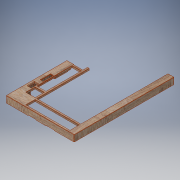
# Autodesk Inventor part: TopCase
Saved by Autodesk Inventor 2018 (Build 220112000, 112)
## iProperties
Created: 2024-10-01
Part Number: TopCase
Material: Wood (Maple)
Document SubType Name: Modeling
Designer: yuchi
Density: 0.67 g/cm^3
Appearance: Oak - Herringbone
Author: yuchi
Autodesk Inventor part; units mm, degrees
ref_plane "YZ Plane" through (0, 0, 0) normal (1, 0, 0) x (0, 1, 0)
sketch "Sketch2" plane through (0, 0, 0) normal (0, 1, 0) x (-1, 0, 0)
  line L0 (12.7, -3.9682) -> (152.454, -3.9682)
  line L1 (119.6499, -137.3179) -> (119.6499, -146.8429)
  line L2 (119.6499, -146.8429) -> (95.8374, -146.8429)
  line L3 (95.8374, -146.8429) -> (95.8374, -156.3679)
  line L4 (95.8374, -156.3679) -> (76.7874, -156.3679)
  line L5 (76.7874, -156.3679) -> (76.7874, -161.1304)
  line L6 (76.7874, -161.1304) -> (57.7374, -161.1304)
  line L7 (57.7374, -161.1304) -> (57.7374, -170.6554)
  line L8 (57.7374, -170.6554) -> (38.6874, -170.6554)
  line L9 (38.6874, -170.6554) -> (38.6874, -223.0434)
  line L10 (12.7, -223.0434) -> (38.6874, -223.0434)
  line L11 (149.794, -46.2682) -> (142.144, -46.2682)
  line L12 (142.144, -46.2682) -> (142.144, -61.4382)
  line L13 (142.144, -61.4382) -> (149.794, -61.4382)
  line L14 (149.794, -61.4382) -> (149.794, -46.2682)
  line L15 (138.7, -32.5419) -> (119.65, -32.5419)
  line L16 (119.65, -32.5419) -> (119.65, -51.5919)
  line L17 (119.65, -51.5919) -> (138.7, -51.5919)
  line L18 (138.7, -51.5919) -> (138.7, -32.5419)
  line L19 (138.7, -56.3549) -> (119.65, -56.3549)
  line L20 (119.65, -56.3549) -> (119.65, -132.5549)
  line L21 (119.65, -132.5549) -> (138.7, -132.5549)
  line L22 (138.7, -132.5549) -> (138.7, -56.3549)
  line L23 (114.887, -32.5434) -> (114.887, -73.9353)
  line L24 (114.887, -73.9353) -> (114.887, -146.8429)
  line L25 (114.887, -32.5434) -> (19.637, -32.5434)
  line L26 (19.637, -32.5434) -> (19.637, -223.0434)
  line L27 (114.887, -27.7804) -> (19.637, -27.7804)
  line L28 (114.887, -27.7804) -> (114.887, -8.7304)
  line L29 (114.887, -8.7304) -> (19.637, -8.7304)
  line L30 (19.637, -8.7304) -> (19.637, -27.7804)
  line L31 (12.7, -3.9682) -> (7.183, -3.9682)
  line L32 (7.183, -223.0434) -> (12.7, -223.0434)
  line L33 (152.454, -3.9682) -> (152.7, -3.9682)
  line L34 (149.195, -71.4432) -> (143.445, -71.4432)
  line L35 (143.445, -71.4432) -> (143.445, -93.9432)
  line L36 (143.445, -93.9432) -> (149.195, -93.9432)
  line L37 (149.195, -93.9432) -> (149.195, -71.4432)
  line L38 (6.2, -3.9682) -> (7.183, -3.9682)
  line L39 (6.2, -3.9682) -> (6.2, -223.0434)
  line L40 (6.2, -223.0434) -> (7.183, -223.0434)
  line L41 (138.932, -51.9234) -> (119.4185, -51.9234)
  line L42 (138.932, -56.0234) -> (119.4185, -56.0234)
  line L43 (119.4185, -56.0234) -> (119.4185, -132.8864)
  line L44 (119.4185, -136.9864) -> (119.65, -136.9864)
  line L45 (119.4185, -136.9864) -> (119.4185, -146.8429)
  line L46 (138.932, -51.9234) -> (138.932, -32.2099)
  line L47 (138.932, -32.2099) -> (130.4516, -32.2099)
  line L48 (130.4516, -32.2099) -> (119.4185, -32.2099)
  line L49 (119.4185, -32.2099) -> (119.4185, -51.9234)
  line L50 (138.932, -56.0234) -> (138.932, -132.8864)
  line L51 (138.932, -132.8864) -> (119.4185, -132.8864)
  line L52 (115.119, -28.1119) -> (19.405, -28.1119)
  line L53 (115.1185, -32.2119) -> (19.405, -32.2119)
  line L54 (19.405, -28.1119) -> (19.405, -8.3984)
  line L55 (115.119, -28.1119) -> (115.119, -8.3984)
  line L56 (115.119, -8.3984) -> (19.405, -8.3984)
  line L57 (115.1185, -32.2119) -> (115.1185, -146.8429)
  line L58 (19.405, -32.2119) -> (19.405, -223.0434)
  line L59 (152.7, -3.9682) -> (154.2, -3.9682)
  line L60 (154.2, -3.9682) -> (154.2, -137.3179)
  line L61 (142.144, -46.2682) -> (142.144, -6.3492)
  line L62 (142.144, -6.3492) -> (12.7, -6.3492)
  line L63 (12.7, -6.3492) -> (12.7, -223.0434)
  line L64 (149.794, -61.4382) -> (152.7, -61.4382)
  line L65 (138.932, -136.9864) -> (138.932, -137.3179)
  line L66 (138.932, -136.9864) -> (119.65, -136.9864)
  line L67 (154.2, -137.3179) -> (119.6499, -137.3179)
  line L68 (138.932, -137.3179) -> (119.4185, -137.3179)
  line L69 (119.4185, -137.3179) -> (119.4185, -136.9864)
  line L70 (119.4185, -136.9864) -> (138.932, -136.9864)
  line L71 (138.932, -136.9864) -> (138.932, -137.3179)
  line L72 (119.4185, -146.8429) -> (119.6499, -146.8429)
  line L73 (119.6499, -146.8429) -> (119.6499, -137.3179)
  line L74 (119.6499, -137.3179) -> (119.4185, -137.3179)
  line L75 (119.4185, -137.3179) -> (119.4185, -146.8429)
  line L76 (119.6499, -146.8429) -> (119.4185, -146.8429)
  line L77 (119.4185, -146.8429) -> (119.4185, -137.3179)
  line L78 (119.4185, -137.3179) -> (119.6499, -137.3179)
  line L79 (119.6499, -137.3179) -> (119.6499, -146.8429)
  line L80 (152.7, -61.4382) -> (152.7, -137.3179)
  line L81 (152.7, -137.3179) -> (138.932, -137.3179)
  line L82 (138.932, -136.9864) -> (138.932, -137.3179)
  line L83 (138.932, -136.9864) -> (119.4185, -136.9864)
  line L84 (119.4185, -136.9864) -> (119.4185, -146.8429)
  line L85 (119.4185, -146.8429) -> (115.1185, -146.8429)
  line L86 (115.1185, -146.8429) -> (115.1185, -32.2119)
  line L87 (115.1185, -32.2119) -> (19.405, -32.2119)
  line L88 (19.405, -32.2119) -> (19.405, -223.0434)
  line L89 (19.405, -223.0434) -> (12.7, -223.0434)
  line L90 (12.7, -223.0434) -> (12.7, -6.3492)
  line L91 (12.548, -6.3492) -> (142.144, -6.3492)
  line L92 (142.144, -6.3492) -> (142.144, -46.2682)
  line L93 (142.144, -46.2682) -> (142.144, -61.4382)
  line L94 (142.144, -61.4382) -> (152.7, -61.4382)
  line L95 (147.054, -137.3179) -> (147.054, -101.4889)
  line L96 (147.054, -101.4889) -> (152.7, -101.4889)
  point P0 (0, 0)
  point P1 (152.454, -6.3489)
  point P2 (127.8231, -53.9734)
  point P3 (117.2685, -47.3899)
  point P4 (128.6114, -134.9364)
  point P5 (108.1778, -30.1619)
  point P6 (150.627, -127.3179)
  point P7 (9.45, -127.3179)
  point P8 (9.45, -212.9184)
  point P9 (9.45, -13.9682)
  point P10 (150.627, -13.9682)
  dimension "d32" = 9.525
  dimension "d33" = 23.8125
  dimension "d34" = 9.525
  dimension "d35" = 19.05
  dimension "d36" = 4.7625
  dimension "d37" = 19.05
  dimension "d38" = 9.525
  dimension "d39" = 19.05
  dimension "d40" = 52.388
  dimension "d45" = 15.17
  dimension "d51" = 19.05
  dimension "d52" = 76.2
  dimension "d53" = 4.763
  dimension "d55" = 4.763
  dimension "d56" = 19.05
  dimension "d60" = 0.246
  dimension "d65" = 10.005
  dimension "d66" = 22.5
  dimension "d68" = 13.754
  dimension "d75" = 5.75
  dimension "d80" = 2.66
  dimension "d82" = 2.3815
  dimension "d83" = 2.3815
  dimension "d84" = 2.05
  dimension "d85" = 2.05
  dimension "d86" = 2.3815
  dimension "d88" = 4.763
  dimension "d89" = 2.15
  dimension "d97" = 0.232
  dimension "d98" = 19.05
  dimension "d99" = 19.05
  dimension "d100" = 0.332
  dimension "d101" = 0.232
  dimension "d102" = 2.3815
  dimension "d103" = 2.05
  dimension "d104" = 2.05
  dimension "d105" = 0.232
  dimension "d106" = 0.232
  dimension "d107" = 0.332
  dimension "d108" = 2.15
  dimension "d109" = 0.232
  dimension "d113" = 1.5
  dimension "d132" = 35.829
  dimension "d144" = 7.146
  dimension "d145" = 3.573
  dimension "d146" = 10
  dimension "d147" = 3.25
  dimension "d149" = 3.25
  dimension "d150" = 3.573
  dimension "d151" = 10
  dimension "d153" = 10.125
  dimension "d157" = 10
  dimension "d158" = 10
  dimension "d180" = 3.25
  dimension "d221" = 130.9681
  dimension "d224" = 43.4216
  dimension "d275" = 4.763
  dimension "d276" = 148
  dimension "d277" = 95.25
  dimension "d278" = 95.25
  dimension "d279" = 190.5
  constraints: 194 end point, 27 perpendicular, 26 horizontal, 22 parallel, 12 vertical, 11 point on line, 6 collinear
  measures "d32" distance of L1.start L1.end
  measures "d33" distance of L1.end L2.end
  measures "d34" distance of L2.end L3.end
  measures "d35" distance of L3.end L4.end
  measures "d36" distance of L4.end L5.end
  measures "d37" distance of L5.end L6.end
  measures "d38" distance of L6.end L7.end
  measures "d39" distance of L7.end L8.end
  measures "d40" distance of L8.end L9.end
  measures "d45" distance between parallel lines of L13 L11
  measures "d51" distance of L20.end L21.end
  measures "d52" distance of L19.end L20.end
  measures "d53" distance between parallel lines of L16 L23
  measures "d55" distance between parallel lines of L27 L25
  measures "d56" distance of L27.start L28.end
  measures "d60" distance of L0.end L33.end
  measures "d65" distance between parallel lines of L13 L34
  measures "d66" distance between parallel lines of L36 L34
  measures "d68" distance from line of point (152.454, -6.349) L18
  measures "d75" distance between parallel lines of L35 L37
  measures "d80" distance from line of point (152.454, -6.349) L14
  measures "d82" distance from line of L17 point (127.823, -53.973)
  measures "d83" distance from line of L19 point (127.823, -53.973)
  measures "d84" distance from line of L41 point (127.823, -53.973)
  measures "d85" distance from line of point (127.823, -53.973) L42
  measures "d86" distance from line of L23 point (117.269, -47.39)
  measures "d88" distance between parallel lines of L20 L23
  measures "d89" distance from line of L43 point (117.269, -47.39)
  measures "d97" distance from line of L41.start L18
  measures "d98" distance between parallel lines of L16 L18
  measures "d99" distance between parallel lines of L17 L15
  measures "d100" distance from line of L15 L46.end
  measures "d101" distance from line of L42.start L22
  measures "d102" distance from line of L25 point (108.178, -30.162)
  measures "d103" distance from line of L52 point (108.178, -30.162)
  measures "d104" distance from line of L53 point (108.178, -30.162)
  measures "d105" distance from line of L30 L52.end
  measures "d106" distance between parallel lines of L55 L28
  measures "d107" distance between parallel lines of L56 L29
  measures "d108" horizontal distance of L53.start point (117.269, -47.39)
  measures "d109" distance between parallel lines of L26 L58
  measures "d113" distance of L33.end L59.end
  measures "d132" distance of L95.start L95.end
  measures "d144" distance between parallel lines of L60 L95
  measures "d145" distance from line of L95 point (150.627, -127.318)
  measures "d146" distance from line of L31 point (9.45, -13.968)
  measures "d147" distance from line of L39 point (9.45, -13.968)
  measures "d149" distance from line of L39 point (9.45, -212.918)
  measures "d150" distance from line of L60 point (150.627, -13.968)
  measures "d151" distance from line of L0 point (150.627, -13.968)
  measures "d153" distance from line of L32 point (9.45, -212.918)
  measures "d157" distance from line of L67 point (150.627, -127.318)
  measures "d158" distance from line of point (9.45, -127.318) L81
  measures "d180" distance from line of L39 point (9.45, -127.318)
  measures "d221" distance from line of point (128.611, -134.936) L33
  measures "d224" distance from line of point (117.269, -47.39) L33
  measures "d275" distance between parallel lines of L16 L28
  measures "d276" distance between parallel lines of L39 L60
  measures "d277" distance between parallel lines of L23 L26
  measures "d278" distance between parallel lines of L30 L28
  measures "d279" distance between parallel lines of L25 L10
extrude "Extrusion5" add sketch "Sketch2" along normal blind 14 contours L0 L33 L59 L60 L67 L80 L64 L14 L11 L61 L62 L63 L32 L40 L39 L38 L31 | L67 L95 L96 L80 | L63 L62 L61 L12 L13 L64 L80 L96 L95 L67 L65 L66 L44 L45 L2 L57 L53 L58 L10 | L67 L68 L45 L44 L66 L65 | L1 L2 L45 L68
extrude "Extrusion6" cut sketch "Sketch2" along normal blind 14 contours L67 L68 L45 L44 L66 L65
extrude "Extrusion7" cut sketch "Sketch2" along normal blind 14 contours L1 L2 L45 L68
extrude "Extrusion8" cut sketch "Sketch2" along normal blind 10.3 contours L67 L95 L96 L80 | L63 L62 L61 L12 L13 L64 L80 L96 L95 L67 L65 L66 L44 L45 L2 L57 L53 L58 L10 | L13 L12 L11 L14 | L18 L17 L16 L15 | L22 L21 L20 L19 | L27 L30 L29 L28 | L37 L36 L35 L34 | L41 L49 L48 L47 L46 | L50 L51 L43 L42 | L52 L54 L56 L55
extrude "Extrusion9" add sketch "Sketch2" along normal blind 10.3 contours L67 L95 L96 L80
sketch "Sketch8" plane through (-154.2, 0, -137.3179) normal (-1, 0, 0) x (0, 0, 1)
  line L0 (0, 0) -> (0, 14) projected
  line L1 (133.3496, 0) -> (0, 0)
  line L2 (0, 0) -> (0, 14)
  line L3 (0, 14) -> (133.3496, 14)
  line L4 (133.3496, 14) -> (133.3496, 0)
  point P0 (137.3179, 0)
  constraints: 8 end point, 2 parallel, 1 horizontal, 1 perpendicular
extrude "Extrusion10" cut sketch "Sketch8" against normal blind 0.268
sketch "Sketch9" plane through (-6.2, 0, -3.9682) normal (1, 0, 0) x (0, 0, -1)
  line L0 (133.3496, 14) -> (0, 14) projected
  line L1 (2.381, 0) -> (219.0751, 0) projected
  line L2 (0, 14) -> (219.0751, 14)
  line L3 (219.0751, 14) -> (219.0751, 0)
  line L4 (219.0751, 0) -> (0, 0)
  line L5 (0, 0) -> (0, 14)
  point P0 (-3.9682, 0)
  constraints: 8 end point, 2 parallel, 1 horizontal, 1 perpendicular
extrude "Extrusion11" cut sketch "Sketch9" against normal blind 0.049
sketch "Sketch10" plane through (-19.405, 14, -223.0434) normal (-1, 0, 0) x (0, 0, 1)
  line L0 (0, 0) -> (190.8315, 0) projected
  line L1 (216.6941, -3.7) -> (0, -3.7) projected
  line L2 (190.8315, 0) -> (0, 0)
  line L3 (0, 0) -> (0, -3.7)
  line L4 (0, -3.7) -> (190.8315, -3.7)
  line L5 (190.8315, -3.7) -> (190.8315, 0)
  point P0 (223.0434, -14)
  constraints: 8 end point, 2 parallel, 1 horizontal, 1 perpendicular
extrude "Extrusion12" cut sketch "Sketch10" against normal blind 0.473
sketch "Sketch11" plane through (-19.405, 14, -28.1119) normal (-1, 0, 0) x (0, 0, 1)
  line L0 (0, -3.7) -> (19.7135, -3.7) projected
  line L1 (19.7135, 0) -> (0, 0)
  line L2 (0, 0) -> (0, -3.7)
  line L3 (0, -3.7) -> (19.7135, -3.7)
  line L4 (19.7135, -3.7) -> (19.7135, 0)
  point P0 (28.1119, -14)
  constraints: 8 end point, 2 parallel, 1 horizontal, 1 perpendicular
extrude "Extrusion13" cut sketch "Sketch11" against normal blind 0.473
hole "Hole1" at (-9.45, 0, -127.3179) at (-9.45, 0, -212.9184) at (-9.45, 0, -13.9682) direction (0, 1, 0) diameter 2 depth 10 tip angle 118
chamfer "Chamfer2" distance 0.5 angle 45 22 edges at (-18.932, 14, -127.6276) (-67.0255, 14, -28.1119) (-67.0253, 14, -32.2119) (-18.932, 14, -18.2551) (-67.0255, 14, -8.3984) (-115.119, 14, -18.2551) (-129.1753, 14, -32.2099) (-138.932, 14, -42.0666) (-119.4185, 14, -42.0666) (-129.1753, 14, -51.9234) (-142.144, 14, -53.8532) (-145.969, 14, -46.2682) (-149.794, 14, -53.8532) (-145.969, 14, -61.4382) (-129.1753, 14, -56.0234) (-138.932, 14, -94.4549) (-119.4185, 14, -94.4549) (-129.1753, 14, -132.8864) (-115.1185, 14, -89.5274) (-129.1753, 14, -136.9864) (-119.4185, 14, -141.9146) (-138.932, 14, -137.1521)
sketch "Sketch13" plane through (-12.7, 0, -6.3492) normal (-1, 0, 0) x (0, 0, 1)
  line L0 (0, 0) -> (0, 10.3) projected
  line L1 (-216.6941, 0) -> (-216.6941, 10.3) projected
  line L2 (0, 10.3) -> (-216.6941, 10.3)
  line L3 (-216.6941, 10.3) -> (-216.6941, 0)
  line L4 (-216.6941, 0) -> (0, 0)
  line L5 (0, 0) -> (0, 10.3)
  point P0 (6.3492, 0)
  constraints: 8 end point, 2 parallel, 1 horizontal, 1 perpendicular
extrude "Extrusion14" cut sketch "Sketch13" against normal blind 0.268
sketch "Sketch14" plane through (-12.432, 0, -6.3492) normal (-1, 0, 0) x (0, 0, 1)
  line L0 (0, 0) -> (-216.6941, 0) projected
  line L1 (0, 10.3) -> (-20, 10.3)
  line L2 (-20, 10.3) -> (-20, 0)
  line L3 (-20, 0) -> (0, 0)
  line L4 (0, 0) -> (0, 10.3)
  line L5 (-216.6941, 10.3) -> (-196.6941, 10.3)
  line L6 (-196.6941, 10.3) -> (-196.6941, 0)
  line L7 (-196.6941, 0) -> (-216.6941, 0)
  line L8 (-216.6941, 0) -> (-216.6941, 10.3)
  line L9 (-216.6941, 10.3) -> (0, 10.3) projected
  line L10 (-100.9681, 10.3) -> (-140.9681, 10.3)
  line L11 (-140.9681, 10.3) -> (-140.9681, 0)
  line L12 (-140.9681, 0) -> (-100.9681, 0)
  line L13 (-100.9681, 0) -> (-100.9681, 10.3)
  line L14 (-20, 10.3) -> (-100.9681, 10.3)
  line L15 (-100.9681, 10.3) -> (-100.9681, 0)
  line L16 (-100.9681, 0) -> (-20, 0)
  line L17 (-20, 0) -> (-20, 10.3)
  line L18 (-140.9681, 10.3) -> (-196.6941, 10.3)
  line L19 (-196.6941, 10.3) -> (-196.6941, 0)
  line L20 (-196.6941, 0) -> (-140.9681, 0)
  line L21 (-140.9681, 0) -> (-140.9681, 10.3)
  point P0 (6.3492, 0)
  dimension "d183" = 20
  dimension "d184" = 20
  dimension "d185" = 75.726
  dimension "d186" = 115.726
  constraints: 40 end point, 10 parallel, 5 horizontal, 5 perpendicular, 4 point on line
  measures "d183" distance of L3.end L2.end
  measures "d184" distance of L6.end L7.end
  measures "d185" distance between parallel lines of L11 L8
  measures "d186" distance between parallel lines of L13 L8
extrude "Extrusion16" cut sketch "Sketch14" against normal blind 3.25 contours L0 L13 L9 L2 | L0 L6 L9 L11
sketch "Sketch16" plane through (0, 0, 0) normal (0, -1, 0) x (1, 0, 0)
  line L0 (-142.144, -35.1182) -> (-146.144, -35.1182)
  line L1 (-146.144, -35.1182) -> (-146.144, -15.1182)
  line L2 (-146.144, -15.1182) -> (-142.144, -15.1182)
  line L3 (-142.144, -15.1182) -> (-142.144, -35.1182)
  line L4 (-153.932, -3.9682) -> (-6.249, -3.9682) projected
  point P0 (0, 0)
  point P1 (-142.144, -46.2682)
  point P2 (-152.932, -3.9682)
  point P3 (-7.249, -3.9683)
  dimension "d195" = 4
  dimension "d196" = 20
  dimension "d197" = 11.15
  constraints: 8 end point, 3 perpendicular, 1 horizontal
  measures "d195" distance of L0.start L0.end
  measures "d196" distance of L0.end L1.end
  measures "d197" distance between parallel lines of L4 L2
extrude "Extrusion17" cut sketch "Sketch16" against normal blind 10.3
fillet "Fillet6" radius 1 1 edges at (-12.432, 5.15, -6.3492)
sketch "Sketch18" plane through (-152.7, 0, -101.4889) normal (0, 0, 1) x (1, 0, 0)
  line L0 (0, 10.3) -> (5.646, 10.3) projected
  line L1 (5.646, 10.3) -> (0, 10.3)
  line L2 (0, 10.3) -> (0, 0)
  line L3 (0, 0) -> (5.646, 0)
  line L4 (5.646, 0) -> (5.646, 10.3)
  point P0 (152.7, 0)
  constraints: 8 end point, 2 parallel, 1 horizontal, 1 perpendicular
extrude "Extrusion18" cut sketch "Sketch18" against normal blind 1
sketch "Sketch19" plane through (-147.054, 0, -137.3179) normal (1, 0, 0) x (0, 0, -1)
  line L0 (0, 10.3) -> (-34.829, 10.3)
  line L1 (-34.829, 10.3) -> (-34.829, 0)
  line L2 (-34.829, 0) -> (0, 0)
  line L3 (0, 0) -> (0, 10.3)
  point P0 (-137.3179, 0)
  constraints: 8 end point, 2 parallel, 1 horizontal, 1 perpendicular
extrude "Extrusion19" add sketch "Sketch19" against normal blind 4
sketch "Sketch20" plane through (0, 0, 0) normal (0, -1, 0) x (1, 0, 0)
  line L0 (-147.054, -137.3179) -> (-153.932, -137.3179) projected
  line L1 (-153.932, -3.9682) -> (-153.932, -137.3179) projected
  line L2 (-153.932, -3.9682) -> (-6.249, -3.9682) projected
  point P0 (0, 0)
  point P1 (-150.432, -127.3179)
  point P2 (-150.432, -13.9682)
  point P3 (-142.932, -137.3179)
  point P4 (-153.932, -4.9682)
  point P5 (-152.932, -3.9682)
  point P6 (-7.249, -3.9683)
  dimension "d236" = 10
  dimension "d237" = 3.5
  dimension "d238" = 3.5
  dimension "d239" = 10
  measures "d236" distance from line of point (-150.432, -127.318) L0
  measures "d237" distance from line of L1 point (-150.432, -127.318)
  measures "d238" distance from line of L1 point (-150.432, -13.968)
  measures "d239" distance from line of L2 point (-150.432, -13.968)
hole "Hole3" at (-150.432, 0, -127.3179) at (-150.432, 0, -13.9682) direction (0, 1, 0) diameter 2 depth 10 tip angle 118
sketch "Sketch21" plane through (0, 0, 0) normal (0, -1, 0) x (1, 0, 0)
  line L0 (-153.932, -3.9682) -> (-153.932, -137.3179) projected
  line L1 (-147.054, -102.4889) -> (-152.7, -102.4889) projected
  line L2 (-6.249, -223.0434) -> (-6.249, -3.9682) projected
  circle A0 centre (-149.932, -122.3179) radius 0.75
  circle A1 centre (-9.95, -122.3179) radius 0.75
  line L3 (-153.932, -3.9682) -> (-6.249, -3.9682) projected
  circle A2 centre (-149.932, -8.9682) radius 0.75
  line L4 (-9.182, -203.0434) -> (-12.432, -203.0434) projected
  circle A3 centre (-9.95, -207.9184) radius 0.75
  line L5 (-147.054, -137.3179) -> (-153.932, -137.3179) projected
  circle A4 centre (-150.432, -127.3179) radius 1 projected
  circle A5 centre (-150.432, -13.9682) radius 1 projected
  circle A6 centre (-9.45, -127.3179) radius 1 projected
  line L6 (-9.182, -107.3174) -> (-12.432, -107.3174) projected
  circle A7 centre (-9.45, -212.9184) radius 1 projected
  point P0 (0, 0)
  point P1 (-153.932, -4.9682)
  point P2 (-149.054, -102.4889)
  point P3 (-6.249, -4.9683)
  point P4 (-152.932, -3.9682)
  point P5 (-7.249, -3.9683)
  point P6 (-10.182, -203.0434)
  point P7 (-11.432, -203.0434)
  point P8 (-10.182, -107.3174)
  point P9 (-11.432, -107.3174)
  dimension "d252" = 1.5
  dimension "d253" = 1.5
  dimension "d255" = 1.5
  dimension "d259" = 1.5
  dimension "d270" = 0.5
  dimension "d273" = 5
  dimension "d274" = 0.5
  dimension "d291" = 0.5
  dimension "d333" = 5
  dimension "d335" = 5
  dimension "d347" = 5
  dimension "d348" = 0.5
  constraints: 8 coincident, 4 centre point
  measures "d252" diameter of A0
  measures "d253" diameter of A1
  measures "d255" diameter of A2
  measures "d259" diameter of A3
  measures "d270" horizontal distance of point (-150.432, -127.318) point (-149.932, -122.318)
  measures "d273" vertical distance of point (-149.932, -8.968) point (-150.432, -13.968)
  measures "d274" horizontal distance of A2.centre point (-150.432, -13.968)
  measures "d291" horizontal distance of point (-9.95, -122.318) point (-9.45, -127.318)
  measures "d333" vertical distance of point (-149.932, -122.318) point (-150.432, -127.318)
  measures "d335" vertical distance of point (-9.45, -127.318) point (-9.95, -122.318)
  measures "d347" vertical distance of point (-9.95, -207.918) point (-9.45, -212.918)
  measures "d348" horizontal distance of A3.centre point (-9.45, -212.918)
hole "Hole4" at (-149.932, 0, -122.3179) at (-9.95, 0, -122.3179) at (-149.932, 0, -8.9682) at (-9.95, 0, -207.9184) direction (0, 1, 0) diameter 2 depth 10 tip angle 118
sketch "Sketch25" plane through (-6.249, 0, -3.9682) normal (1, 0, 0) x (0, 0, -1)
  line L0 (3.381, 0) -> (219.0751, 0) projected
  line L1 (0, 14) -> (0, 0) projected
  line L2 (219.0751, 0) -> (0, 0)
  line L3 (0, 0) -> (0, 14)
  line L4 (0, 14) -> (219.0751, 14)
  line L5 (219.0751, 14) -> (219.0751, 0)
  point P0 (-3.9682, 0)
  point P1 (200.0751, 0)
  constraints: 8 end point, 2 parallel, 1 horizontal, 1 perpendicular
extrude "Extrusion20" add sketch "Sketch25" along normal blind 0.817
sketch "Sketch27" plane through (-147.054, 0, -137.3179) normal (1, 0, 0) x (0, 0, -1)
  line L0 (-34.829, 10.3) -> (0, 10.3) projected
  line L1 (-34.829, 10.3) -> (-34.829, 0) projected
  line L2 (0, 10.3) -> (-34.829, 10.3)
  line L3 (-34.829, 10.3) -> (-34.829, 0)
  line L4 (-34.829, 0) -> (0, 0)
  line L5 (0, 0) -> (0, 10.3)
  point P0 (-137.3179, 0)
  constraints: 8 end point, 2 parallel, 1 horizontal, 1 perpendicular
extrude "Extrusion21" cut sketch "Sketch27" against normal blind 1.378
sketch "Sketch33" plane through (-153.932, 0, -137.3179) normal (-1, 0, 0) x (0, 0, 1)
  line L0 (0, 14) -> (133.3496, 14) projected
  line L1 (0, 10.3) -> (0, 0) projected
  line L2 (133.3496, 14) -> (0, 14)
  line L3 (0, 14) -> (0, 0)
  line L4 (0, 0) -> (133.3496, 0)
  line L5 (133.3496, 0) -> (133.3496, 14)
  point P0 (137.3179, 0)
  constraints: 8 end point, 2 parallel, 1 horizontal, 1 perpendicular
extrude "Extrusion26" add sketch "Sketch33" along normal blind 1
ref_plane "Work Plane5" through (-153.932, 13.5, -3.9682) normal (0, 0, 1) x (1, 0, 0)
sketch "Sketch34" plane through (-153.932, 13.5, -3.9682) normal (0, 0, 1) x (1, 0, 0)
  line L0 (148.5, -13.5) -> (148.5, 0) projected
  line L1 (-1, -13.5) -> (148.5, -13.5) projected
  arc A0 (89.129, -12.466) -> (89.129, -19.566) centre (89.129, -16.016) ccw
  arc A1 (103.149, -19.566) -> (103.149, -12.466) centre (103.149, -16.016) ccw
  line L2 (89.129, -12.466) -> (103.149, -12.466)
  line L3 (103.149, -19.566) -> (89.129, -19.566)
  arc A2 (63.269, -19.566) -> (63.269, -12.466) centre (63.269, -16.016) ccw
  arc A3 (49.249, -12.466) -> (49.249, -19.566) centre (49.249, -16.016) ccw
  line L4 (49.249, -19.566) -> (63.269, -19.566)
  line L5 (63.269, -12.466) -> (49.249, -12.466)
  point P0 (153.932, -13.5)
  point P1 (96.139, -16.016)
  point P2 (0, -13.5)
  point P3 (147.5, -13.5)
  point P4 (56.259, -16.016)
  dimension "d315" = 2.516
  dimension "d316" = 52.361
  dimension "d317" = 39.88
  dimension "d318" = 2.516
  dimension "d319" = 7.01
  dimension "d320" = 7.01
  dimension "d321" = 7.01
  dimension "d322" = 7.01
  dimension "d323" = 3.55
  dimension "d324" = 3.55
  dimension "d325" = 3.55
  dimension "d326" = 3.55
  dimension "d327" = 7.1
  dimension "d328" = 7.1
  constraints: 8 end point, 8 point on circle, 4 centre point, 4 coincident, 4 horizontal alignment, 2 horizontal, 2 parallel, 1 tangent
  measures "d315" distance from line of L1 point (96.139, -16.016)
  measures "d316" distance from line of L0 point (96.139, -16.016)
  measures "d317" distance of point (96.139, -16.016) point (56.259, -16.016)
  measures "d318" distance from line of L1 point (56.259, -16.016)
  measures "d319" distance of point (63.269, -16.016) point (56.259, -16.016)
  measures "d320" distance of point (56.259, -16.016) point (49.249, -16.016)
  measures "d321" distance of point (96.139, -16.016) point (89.129, -16.016)
  measures "d322" distance of point (103.149, -16.016) point (96.139, -16.016)
  measures "d323" radius of A0
  measures "d324" radius of A1
  measures "d325" radius of A2
  measures "d326" radius of A3
  measures "d327" distance between parallel lines of L4 L5
  measures "d328" distance between parallel lines of L2 L3
extrude "Extrusion27" cut sketch "Sketch34" against normal blind 10
sketch "Sketch35" plane through (-138.932, 10.3, -137.3179) normal (0, 0, -1) x (-1, 0, 0)
  line L0 (9.5, -10.3) -> (16, -10.3) projected
  line L1 (16, 3.7) -> (16, -10.3) projected
  line L2 (10.862, -10.3) -> (3.212, -10.3) projected
  line L3 (3.212, -10.3) -> (-125.5, -10.3) projected
  arc A0 (11.6009, -10.3) -> (9.232, -9.394) centre (9.232, -12.944) ccw
  line L4 (2.212, -10.3) -> (3.212, -10.3) projected
  line L5 (11.6009, -10.3) -> (2.212, -10.3)
  line L6 (9.232, -9.394) -> (2.212, -9.394)
  line L7 (2.212, 0) -> (2.212, -10.3) projected
  line L8 (2.212, -10.3) -> (2.212, -9.394)
  point P0 (-138.932, -10.3)
  point P1 (2.222, -12.944)
  point P2 (16, 3.2)
  point P3 (4.212, -10.3)
  point P4 (-32.0237, -10.3)
  point P5 (-50.4943, -10.3)
  dimension "d336" = 2.644
  dimension "d337" = 13.778
  dimension "d338" = 7.01
  dimension "d342" = 3.55
  dimension "d343" = 3.55
  constraints: 6 end point, 2 collinear, 2 point on circle, 1 centre point, 1 coincident, 1 horizontal, 1 point on line
  measures "d336" distance from line of L0 point (2.222, -12.944)
  measures "d337" distance from line of L1 point (2.222, -12.944)
  measures "d338" distance of point (9.232, -12.944) point (2.222, -12.944)
  measures "d342" radius of A0
  measures "d343" distance from line of point (2.222, -12.944) L6
extrude "Extrusion28" cut sketch "Sketch35" against normal blind 6
sketch "Sketch37" plane through (0, 0, 0) normal (0, -1, 0) x (1, 0, 0)
  line L0 (-12.432, -7.3492) -> (-12.432, -5.9682)
  line L1 (-48.6007, -5.9682) -> (-13.432, -5.9682) projected
  line L2 (-12.432, -5.9682) -> (-13.432, -5.9682)
  line L3 (-13.432, -5.9682) -> (-13.432, -7.3492)
  line L4 (-13.432, -7.3492) -> (-12.432, -7.3492)
  line L5 (-141.144, -6.3493) -> (-141.144, -5.9682) projected
  line L6 (-141.144, -5.9682) -> (-141.144, -7.3492)
  line L7 (-142.144, -15.1182) -> (-142.144, -6.3492) projected
  line L8 (-141.144, -7.3492) -> (-142.144, -7.3492)
  line L9 (-142.144, -7.3492) -> (-142.144, -5.9682)
  line L10 (-142.144, -5.9682) -> (-141.144, -5.9682)
  point P0 (0, 0)
  point P1 (-142.144, -14.1182)
  constraints: 16 end point, 5 perpendicular, 2 collinear, 2 point on line, 1 vertical
extrude "Extrusion30" cut sketch "Sketch37" against normal up to surface (10.3 mm away)
sketch "Sketch38" plane through (-149.794, 0, -61.4382) normal (0, 0, -1) x (-1, 0, 0)
  line L0 (2.906, 10.3) -> (0, 10.3) projected
  line L1 (2.906, 0) -> (0, 0) projected
  line L2 (2.906, 10.3) -> (0, 10.3)
  line L3 (0, 10.3) -> (0, 0)
  line L4 (0, 0) -> (2.906, 0)
  line L5 (2.906, 0) -> (2.906, 10.3)
  point P0 (-149.794, 0)
  constraints: 8 end point, 2 parallel, 1 horizontal, 1 perpendicular
extrude "Extrusion31" cut sketch "Sketch38" against normal blind 0.5
sketch "Sketch39" plane through (0, 14, 0) normal (0, 1, 0) x (1, 0, 0)
  line L0 (-149.609, 46.5182) -> (-142.329, 46.5182)
  line L1 (-142.329, 46.5182) -> (-142.329, 61.1882)
  line L2 (-142.329, 61.1882) -> (-149.609, 61.1882)
  line L3 (-149.609, 61.1882) -> (-149.609, 46.5182)
  line L4 (-150.294, 45.7682) -> (-141.644, 45.7682) projected
  line L5 (-142.144, 61.4382) -> (-142.144, 46.2682) projected
  line L6 (-149.794, 46.2682) -> (-149.794, 61.4382) projected
  line L7 (-149.794, 61.4382) -> (-142.144, 61.4382) projected
  line L8 (-150.294, 61.9382) -> (-150.294, 45.7682) projected
  line L9 (-150.294, 61.9382) -> (-141.644, 61.9382)
  line L10 (-141.644, 61.9382) -> (-141.644, 45.7682)
  line L11 (-141.644, 45.7682) -> (-150.294, 45.7682)
  line L12 (-150.294, 45.7682) -> (-150.294, 61.9382)
  point P0 (0, 0)
  dimension "d356" = 0.75
  dimension "d357" = 0.185
  dimension "d358" = 0.185
  dimension "d359" = 0.25
  constraints: 16 end point, 4 parallel, 2 horizontal, 2 perpendicular
  measures "d356" distance between parallel lines of L0 L4
  measures "d357" distance between parallel lines of L5 L1
  measures "d358" distance between parallel lines of L3 L6
  measures "d359" distance between parallel lines of L7 L2
extrude "Extrusion32" add sketch "Sketch39" against normal up to surface (3.7 mm away)
chamfer "Chamfer7" distance 1 angle 45 4 edges at (-145.969, 14, -61.1882) (-149.609, 14, -53.8532) (-142.329, 14, -53.8532) (-145.969, 14, -46.5182)
sketch "Sketch40" plane through (0, 14, 0) normal (0, 1, 0) x (1, 0, 0)
  line L0 (-139.432, 52.4234) -> (-139.432, 31.7099) projected
  line L1 (-139.432, 52.2239) -> (-118.9185, 52.2239)
  line L2 (-118.9185, 31.7099) -> (-118.9185, 52.4234) projected
  line L3 (-139.432, 31.7099) -> (-118.9185, 31.7099) projected
  line L4 (-118.9185, 52.4234) -> (-139.432, 52.4234) projected
  line L5 (-139.432, 52.2239) -> (-118.9185, 52.2239)
  line L6 (-118.9185, 52.2239) -> (-118.9185, 52.4234)
  line L7 (-118.9185, 52.4234) -> (-139.432, 52.4234)
  line L8 (-139.432, 52.4234) -> (-139.432, 52.2239)
  point P0 (0, 0)
  dimension "d365" = 20.514
  constraints: 10 end point, 2 horizontal, 2 parallel, 2 point on line, 1 perpendicular
  measures "d365" distance between parallel lines of L3 L1
extrude "Extrusion33" add sketch "Sketch40" against normal up to surface (3.7 mm away) contours L4 L2 L1 L0
sketch "Sketch41" plane through (0, 14, 0) normal (0, 1, 0) x (1, 0, 0)
  line L0 (-138.932, 32.2099) -> (-138.932, 51.9234) projected
  line L1 (-119.4185, 51.9234) -> (-119.4185, 32.2099) projected
  line L2 (-138.932, 32.2099) -> (-119.4185, 32.2099)
  line L3 (-119.4185, 32.2099) -> (-119.4185, 51.7239)
  line L4 (-119.4185, 51.7239) -> (-138.932, 51.7239)
  line L5 (-138.932, 51.7239) -> (-138.932, 32.2099)
  line L6 (-139.2325, 52.2239) -> (-139.432, 52.2239) projected
  line L7 (-118.9185, 31.7099) -> (-118.9185, 52.2239) projected
  line L8 (-139.432, 52.2239) -> (-118.9185, 52.2239)
  line L9 (-118.9185, 52.2239) -> (-119.4185, 51.7239)
  line L10 (-138.932, 51.7239) -> (-139.432, 52.2239)
  point P0 (0, 0)
  dimension "d368" = 19.514
  constraints: 14 end point, 2 horizontal, 2 parallel, 1 perpendicular, 1 point on line
  measures "d368" distance between parallel lines of L4 L2
extrude "Extrusion34" add sketch "Sketch41" against normal up to surface (3.7 mm away) contours L10 L6 L8 L9 L4
chamfer "Chamfer8" distance 0.5 angle 45 1 edges at (-129.1753, 14, -51.7239)
sketch "Sketch42" plane through (0, 10.3, 0) normal (0, -1, 0) x (1, 0, 0)
  line L0 (-150.5884, -69.1085) -> (-141.7481, -69.1085)
  line L1 (-141.7481, -69.1085) -> (-141.7481, -97.0438)
  line L2 (-141.7481, -97.0438) -> (-150.5884, -97.0438)
  line L3 (-150.5884, -97.0438) -> (-150.5884, -69.1085)
  point P0 (0, 0)
  constraints: 8 end point, 2 parallel, 1 horizontal, 1 perpendicular
sketch "Sketch43" plane through (-12.432, 0, -6.3492) normal (-1, 0, 0) x (0, 0, 1)
  line L0 (-216.6941, 10.3) -> (-196.6941, 10.3) projected
  line L1 (0.381, 0) -> (0.381, 10.3) projected
  line L2 (-216.6941, 10.3) -> (0.381, 10.3)
  line L3 (0.381, 10.3) -> (0.381, 0)
  line L4 (0.381, 0) -> (-216.6941, 0)
  line L5 (-216.6941, 0) -> (-216.6941, 10.3)
  point P0 (6.3492, 0)
  constraints: 8 end point, 2 parallel, 1 horizontal, 1 perpendicular
extrude "Extrusion35" cut sketch "Sketch43" against normal blind 0.1
sketch "Sketch44" plane through (-142.144, 0, -46.2682) normal (1, 0, 0) x (0, 0, -1)
  line L0 (0, 10.3) -> (-11.15, 10.3) projected
  line L1 (-11.15, 10.3) -> (-11.15, 0) projected
  line L2 (0, 10.3) -> (-11.15, 10.3)
  line L3 (-11.15, 10.3) -> (-11.15, 0)
  line L4 (-11.15, 0) -> (0, 0)
  line L5 (0, 0) -> (0, 10.3)
  line L6 (-40.3, 10.3) -> (-31.15, 10.3) projected
  line L7 (-39.919, 0) -> (-39.919, 10.3) projected
  line L8 (-31.15, 10.3) -> (-39.919, 10.3)
  line L9 (-39.919, 10.3) -> (-39.919, 0)
  line L10 (-39.919, 0) -> (-31.15, 0)
  line L11 (-31.15, 0) -> (-31.15, 10.3)
  point P0 (-46.2682, 0)
  constraints: 16 end point, 4 parallel, 2 horizontal, 2 perpendicular
extrude "Extrusion36" cut sketch "Sketch44" against normal blind 0.1
sketch "Sketch45" plane through (-141.144, 0, -5.9682) normal (0, 0, -1) x (-1, 0, 0)
  line L0 (0, 10.3) -> (1, 10.3) projected
  line L1 (1, 10.3) -> (0, 10.3)
  line L2 (0, 10.3) -> (0, 0)
  line L3 (0, 0) -> (1, 0)
  line L4 (1, 0) -> (1, 10.3)
  point P0 (-141.144, 0)
  constraints: 8 end point, 2 parallel, 1 horizontal, 1 perpendicular
extrude "Extrusion37" add sketch "Sketch45" along normal up to surface (0.381 mm away)
fillet "Fillet19" radius 1 6 edges at (-142.244, 5.15, -46.2682) (-149.794, 5.15, -60.9382) (-142.244, 5.15, -35.1182) (-146.144, 5.15, -35.1182) (-146.144, 5.15, -15.1182) (-142.244, 5.15, -15.1182)
sketch "Sketch46" plane through (-18.932, 10.3, -223.0434) normal (0, 0, -1) x (-1, 0, 0)
  line L0 (-6.6, -10.3) -> (-6.6, 0) projected
  line L1 (-6.6, 0) -> (0, 0) projected
  line L2 (0, 0) -> (0, 3.2) projected
  line L3 (-0.5, 3.7) -> (0, 3.2) projected
  line L4 (-13.5, 3.7) -> (-0.5, 3.7) projected
  line L5 (-13.5, -10.3) -> (-13.5, 3.7) projected
  line L6 (-13.5, -10.3) -> (-6.6, -10.3) projected
  point P0 (-18.932, -10.3)
extrude "Extrusion38" cut sketch "Sketch46" against normal blind 0.125
sketch "Sketch47" plane through (-115.1185, 10.3, -146.8429) normal (0, 0, -1) x (-1, 0, 0)
  line L0 (3.8, 3.7) -> (4.3, 3.2) projected
  line L1 (0.5, 3.7) -> (3.8, 3.7) projected
  line L2 (0, 3.2) -> (0.5, 3.7) projected
  line L3 (0, 0) -> (0, 3.2) projected
  line L4 (0, 0) -> (4.3, 0) projected
  line L5 (4.3, 0) -> (4.3, 3.2) projected
  point P0 (-115.1185, -10.3)
extrude "Extrusion39" cut sketch "Sketch47" against normal blind 0.125
sketch "Sketch48" plane through (-138.932, 10.3, -137.3179) normal (0, 0, -1) x (-1, 0, 0)
  line L0 (11.6009, -10.3) -> (16, -10.3) projected
  line L1 (16, 3.7) -> (16, -10.3) projected
  line L2 (0.5, 3.7) -> (16, 3.7) projected
  line L3 (0, 3.2) -> (0.5, 3.7) projected
  line L4 (0, 3.2) -> (0, 0) projected
  line L5 (0, 0) -> (9.5, 0) projected
  line L6 (9.5, 0) -> (9.5, -9.4041) projected
  arc A0 (11.6009, -10.3) -> (9.5, -9.4041) centre (9.232, -12.944) ccw projected
  point P0 (-138.932, -10.3)
extrude "Extrusion40" cut sketch "Sketch48" against normal blind 0.148
sketch "Sketch49" plane through (-138.932, 10.3, -137.1699) normal (0, 0, -1) x (-1, 0, 0)
  line L0 (9.5, -10.3) -> (9.5, 0) projected
  line L1 (9.5, -10.3) -> (13.5935, -10.3)
  line L2 (13.5935, -10.3) -> (13.5935, -8.1067)
  line L3 (13.5935, -8.1067) -> (9.5, -8.1067)
  line L4 (9.5, -8.1067) -> (9.5, -10.3)
  point P0 (-138.932, -10.3)
  constraints: 8 end point, 2 parallel, 1 horizontal, 1 perpendicular
extrude "Extrusion41" cut sketch "Sketch49" along normal blind 1
sketch "Sketch50" plane through (-67.3074, 0, -6.3492) normal (0, 0, -1) x (-1, 0, 0)
  line L0 (-53.8754, 10.3) -> (74.9366, 10.3) projected
  line L1 (-53.8754, 0) -> (-53.8754, 10.3) projected
  line L2 (-19.0289, 0) -> (-53.8754, 0) projected
  line L3 (74.9366, 0) -> (74.9366, 10.3) projected
  arc A0 (-16.5244, 1.034) -> (-19.0289, 0) centre (-16.5244, -2.516) ccw projected
  line L4 (-16.5244, 1.034) -> (-2.5044, 1.034) projected
  arc A1 (0, 0) -> (-2.5044, 1.034) centre (-2.5044, -2.516) ccw projected
  line L5 (20.8511, 0) -> (0, 0) projected
  arc A2 (23.3556, 1.034) -> (20.8511, 0) centre (23.3556, -2.516) ccw projected
  line L6 (23.3556, 1.034) -> (37.3756, 1.034) projected
  arc A3 (39.88, 0) -> (37.3756, 1.034) centre (37.3756, -2.516) ccw projected
  line L7 (74.9366, 0) -> (39.88, 0) projected
  point P0 (-67.3074, 0)
extrude "Extrusion42" cut sketch "Sketch50" against normal blind 0.124
sketch "Sketch51" plane through (-13.432, 0, -5.9682) normal (0, 0, -1) x (-1, 0, 0)
  line L0 (-1.1, 10.3) -> (0, 10.3) projected
  line L1 (-1.1, 10.3) -> (-1.1, 0) projected
  line L2 (0, 0) -> (-1.1, 0) projected
  line L3 (0, 0) -> (0, 10.3) projected
  point P0 (-13.432, 0)
extrude "Extrusion43" add sketch "Sketch51" along normal up to surface (0.257 mm away)
fillet "Fillet20" radius 1 2 edges at (-12.332, 5.15, -6.2252) (-142.244, 5.15, -6.2252)
sketch "Sketch52" plane through (0, 10.3, 0) normal (0, -1, 0) x (1, 0, 0)
  line L0 (-149.195, -93.9432) -> (-143.445, -93.9432) projected
  line L1 (-149.195, -93.9432) -> (-143.445, -93.9432)
  line L2 (-143.445, -93.9432) -> (-143.445, -71.4432)
  line L3 (-143.445, -71.4432) -> (-149.195, -71.4432)
  line L4 (-149.195, -71.4432) -> (-149.195, -93.9432)
  arc A0 (-141.244, -6.2252) -> (-142.244, -7.2252) centre (-141.244, -7.2252) ccw projected
  line L5 (-142.244, -7.2252) -> (-142.244, -14.1182) projected
  arc A1 (-143.244, -15.1182) -> (-142.244, -14.1182) centre (-143.244, -14.1182) ccw projected
  line L6 (-145.144, -15.1182) -> (-143.244, -15.1182) projected
  arc A2 (-145.144, -15.1182) -> (-146.144, -16.1182) centre (-145.144, -16.1182) ccw projected
  line L7 (-146.144, -34.1182) -> (-146.144, -16.1182) projected
  arc A3 (-146.144, -34.1182) -> (-145.144, -35.1182) centre (-145.144, -34.1182) ccw projected
  line L8 (-143.244, -35.1182) -> (-145.144, -35.1182) projected
  arc A4 (-142.244, -36.1182) -> (-143.244, -35.1182) centre (-143.244, -36.1182) ccw projected
  line L9 (-142.244, -36.1182) -> (-142.244, -45.2682) projected
  arc A5 (-143.244, -46.2682) -> (-142.244, -45.2682) centre (-143.244, -45.2682) ccw projected
  line L10 (-149.794, -46.2682) -> (-143.244, -46.2682) projected
  line L11 (-149.794, -59.9382) -> (-149.794, -46.2682) projected
  arc A6 (-150.794, -60.9382) -> (-149.794, -59.9382) centre (-150.794, -59.9382) ccw projected
  line L12 (-150.794, -60.9382) -> (-152.7, -60.9382) projected
  line L13 (-152.7, -102.4889) -> (-152.7, -60.9382) projected
  line L14 (-152.7, -102.4889) -> (-148.432, -102.4889) projected
  line L15 (-148.432, -102.4889) -> (-148.432, -137.1699) projected
  line L16 (-148.432, -137.1699) -> (-138.932, -137.1699) projected
  line L17 (-138.932, -136.9864) -> (-138.932, -137.1699) projected
  line L18 (-119.4185, -136.9864) -> (-138.932, -136.9864) projected
  line L19 (-119.4185, -146.7179) -> (-119.4185, -136.9864) projected
  line L20 (-119.4185, -146.7179) -> (-115.1185, -146.7179) projected
  line L21 (-115.1185, -32.2119) -> (-115.1185, -146.7179) projected
  line L22 (-18.932, -32.2119) -> (-115.1185, -32.2119) projected
  line L23 (-18.932, -32.2119) -> (-18.932, -222.9184) projected
  line L24 (-18.932, -222.9184) -> (-12.332, -222.9184) projected
  line L25 (-12.332, -222.9184) -> (-12.332, -203.0434) projected
  line L26 (-12.332, -203.0434) -> (-9.182, -203.0434) projected
  line L27 (-9.182, -203.0434) -> (-9.182, -147.3174) projected
  line L28 (-12.332, -147.3174) -> (-9.182, -147.3174) projected
  line L29 (-12.332, -147.3174) -> (-12.332, -107.3174) projected
  line L30 (-12.332, -107.3174) -> (-9.182, -107.3174) projected
  line L31 (-9.182, -107.3174) -> (-9.182, -26.3492) projected
  line L32 (-12.332, -26.3492) -> (-9.182, -26.3492) projected
  line L33 (-12.332, -26.3492) -> (-12.332, -7.2252) projected
  arc A7 (-12.332, -7.2252) -> (-13.332, -6.2252) centre (-13.332, -7.2252) ccw projected
  line L34 (-13.332, -6.2252) -> (-141.244, -6.2252) projected
  line L35 (-18.932, -28.1119) -> (-115.119, -28.1119) projected
  line L36 (-115.119, -8.3984) -> (-115.119, -28.1119) projected
  line L37 (-18.932, -8.3984) -> (-115.119, -8.3984) projected
  line L38 (-18.932, -8.3984) -> (-18.932, -28.1119) projected
  line L39 (-138.932, -56.0234) -> (-138.932, -132.8864) projected
  line L40 (-119.4185, -56.0234) -> (-138.932, -56.0234) projected
  line L41 (-119.4185, -132.8864) -> (-119.4185, -56.0234) projected
  line L42 (-138.932, -132.8864) -> (-119.4185, -132.8864) projected
  line L43 (-149.195, -71.4432) -> (-149.195, -93.9432) projected
  line L44 (-143.445, -71.4432) -> (-149.195, -71.4432) projected
  line L45 (-143.445, -93.9432) -> (-143.445, -71.4432) projected
  line L46 (-149.195, -93.9432) -> (-143.445, -93.9432) projected
  line L47 (-142.329, -46.5182) -> (-142.329, -61.1882) projected
  line L48 (-142.329, -61.1882) -> (-149.609, -61.1882) projected
  line L49 (-149.609, -61.1882) -> (-149.609, -46.5182) projected
  line L50 (-149.609, -46.5182) -> (-142.329, -46.5182) projected
  line L51 (-138.932, -32.2099) -> (-138.932, -51.7239) projected
  line L52 (-119.4185, -32.2099) -> (-138.932, -32.2099) projected
  line L53 (-119.4185, -51.7239) -> (-119.4185, -32.2099) projected
  line L54 (-119.4185, -51.7239) -> (-138.932, -51.7239) projected
  line L55 (-142.329, -61.1882) -> (-138.932, -61.1882)
  line L56 (-138.932, -61.1882) -> (-138.932, -102.4889)
  line L57 (-138.932, -56.0234) -> (-138.932, -132.8864) projected
  line L58 (-149.432, -102.4889) -> (-138.932, -102.4889)
  arc A8 (-150.794, -60.9382) -> (-149.794, -59.9382) centre (-150.794, -59.9382) ccw projected
  line L59 (-150.794, -60.9382) -> (-149.609, -60.9382)
  line L60 (-149.609, -46.5182) -> (-149.609, -61.1882) projected
  point P0 (0, 0)
  constraints: 16 end point, 3 perpendicular, 3 point on line, 2 horizontal, 2 parallel
extrude "Extrusion44" cut sketch "Sketch52" against normal blind 1.86 contours L49 L50 L47 L48
ref_plane "Work Plane4" through (-154.932, 13.5, -3.9682) normal (0, 0, 1) x (1, 0, 0)
sketch "Sketch54" plane through (-5.432, 0, -3.9683) normal (0, 0, 1) x (1, 0, 0)
  arc A0 (-42.8466, 0) -> (-45.351, 1.034) centre (-45.351, -2.516) ccw projected
  line L0 (-42.8466, 0) -> (0, 0) projected
  line L1 (0, 14) -> (0, 0) projected
  line L2 (-149.5, 14) -> (0, 14) projected
  line L3 (-149.5, 0) -> (-149.5, 14) projected
  line L4 (-149.5, 0) -> (-101.7554, 0) projected
  arc A1 (-99.251, 1.034) -> (-101.7554, 0) centre (-99.251, -2.516) ccw projected
  line L5 (-99.251, 1.034) -> (-85.231, 1.034) projected
  arc A2 (-82.7266, 0) -> (-85.231, 1.034) centre (-85.231, -2.516) ccw projected
  line L6 (-82.7266, 0) -> (-61.8754, 0) projected
  arc A3 (-59.371, 1.034) -> (-61.8754, 0) centre (-59.371, -2.516) ccw projected
  line L7 (-59.371, 1.034) -> (-45.351, 1.034) projected
  point P0 (5.432, 0)
extrude "Extrusion45" cut sketch "Sketch54" against normal blind 0.076
sketch "Sketch55" plane through (-148.432, 0, -137.3179) normal (1, 0, 0) x (0, 0, -1)
  line L0 (-0.148, 0.8959) -> (-0.148, 10.3) projected
  line L1 (-34.829, 10.3) -> (-0.148, 10.3) projected
  line L2 (-34.829, 0) -> (-34.829, 10.3) projected
  line L3 (-6, 0) -> (-34.829, 0) projected
  line L4 (-6, 0) -> (-6, 0.8959) projected
  line L5 (-6, 0.8959) -> (-0.148, 0.8959) projected
  point P0 (-137.3179, 0)
extrude "Extrusion46" add sketch "Sketch55" along normal blind 1.8
fillet "Fillet21" radius 2 2 edges at (-146.632, 5.15, -102.4889) (-152.7, 5.15, -102.4889)
chamfer "Chamfer9" distance 0.5 angle 45 3 edges at (-5.432, 14, -113.4813) (-80.182, 14, -4.0443) (-154.932, 14, -70.6071)
fillet "Fillet22" radius 1 2 edges at (-5.432, 6.75, -4.0443) (-154.932, 6.75, -4.0442)
sketch "Sketch57" plane through (0, 10.3, 0) normal (0, -1, 0) x (1, 0, 0)
  line L0 (-149.195, -93.9432) -> (-143.445, -93.9432) projected
  line L1 (-149.195, -93.9432) -> (-143.445, -93.9432)
  line L2 (-143.445, -93.9432) -> (-143.445, -71.4432)
  line L3 (-143.445, -71.4432) -> (-149.195, -71.4432)
  line L4 (-149.195, -71.4432) -> (-149.195, -93.9432)
  point P0 (0, 0)
  constraints: 8 end point, 2 parallel, 1 horizontal, 1 perpendicular
extrude "Extrusion47" add sketch "Sketch57" against normal up to surface (3.7 mm away)
sketch "Sketch58" plane through (0, 14, 0) normal (0, 1, 0) x (1, 0, 0)
  line L0 (-147.017, 71.5802) -> (-141.497, 71.5802)
  line L1 (-141.497, 71.5802) -> (-141.497, 93.9602)
  line L2 (-141.497, 93.9602) -> (-147.017, 93.9602)
  line L3 (-147.017, 93.9602) -> (-147.017, 71.5802)
  line L4 (-142.329, 61.1882) -> (-142.329, 46.5182) projected
  line L5 (-139.432, 137.1699) -> (-154.432, 137.1699) projected
  line L6 (-154.932, 137.1699) -> (-154.932, 5.0442) projected
  line L7 (-138.932, 56.0234) -> (-138.932, 132.8864) projected
  point P0 (0, 0)
  point P1 (-142.329, 53.8532)
  dimension "d411" = 22.38
  dimension "d413" = 5.52
  dimension "d414" = 40.107
  dimension "d416" = 2.565
  constraints: 8 end point, 2 parallel, 1 horizontal, 1 midpoint, 1 perpendicular
  measures "d411" distance between parallel lines of L2 L0
  measures "d413" distance of L1.end L2.end
  measures "d414" distance from line of L2 point (-142.329, 53.853)
  measures "d416" distance between parallel lines of L7 L1
extrude "Extrusion48" cut sketch "Sketch58" against normal through all
sketch "Sketch59" plane through (0, 10.3, 0) normal (0, -1, 0) x (1, 0, 0)
  line L0 (-139.137, -62.5602) -> (-151.537, -62.5602)
  line L1 (-151.537, -62.5602) -> (-151.537, -101.1602)
  line L2 (-151.537, -101.1602) -> (-139.137, -101.1602)
  line L3 (-139.137, -101.1602) -> (-139.137, -62.5602)
  line L4 (-141.497, -93.9602) -> (-147.017, -93.9602) projected
  line L5 (-147.017, -93.9602) -> (-147.017, -71.5802) projected
  line L6 (-141.497, -71.5802) -> (-141.497, -93.9602) projected
  point P0 (0, 0)
  dimension "d419" = 7.2
  dimension "d420" = 38.6
  dimension "d421" = 12.4
  dimension "d423" = 2.36
  constraints: 8 end point, 2 parallel, 1 horizontal, 1 perpendicular
  measures "d419" distance between parallel lines of L2 L4
  measures "d420" distance of L2.end L0.start
  measures "d421" distance of L0.start L0.end
  measures "d423" distance between parallel lines of L3 L6
extrude "Extrusion49" cut sketch "Sketch59" against normal blind 2.2
chamfer "Chamfer10" distance 0.5 angle 45 4 edges at (-144.257, 14, -71.5802) (-147.017, 14, -82.7702) (-141.497, 14, -82.7702) (-144.257, 14, -93.9602)
body "Solid3"
